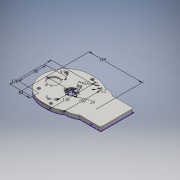
# Autodesk Inventor part: AZ-FLDIC-FWup bottom adapter
Saved by Autodesk Inventor 2016 (Build 200138000, 138)
## iProperties
Created: 2015-08-14
Part Number: AZ-FLDIC-FWup bottom adapter
Material: Generic
Document SubType Name: Modeling
Designer: kthorn
Density: 1 g/cm^3
Appearance: Default
Author: kthorn
Autodesk Inventor part; units mm, degrees
note: some values were not read from the file. Chosen so that the rebuilt part matches the saved one: sketch regions of "Extrusion4".
ref_plane "YZ Plane" through (0, 0, 0) normal (1, 0, 0) x (0, 1, 0)
ref_plane "XZ Plane" through (0, 0, 0) normal (0, 1, 0) x (-1, 0, 0)
ref_plane "XY Plane" through (0, 0, 0) normal (0, 0, 1) x (1, 0, 0)
sketch "Sketch1" plane through (0, 0, 0) normal (0, 0, 1) x (1, 0, 0)
  line L0 (-19.2849, 35) -> (-19.2849, -35) construction
  line L1 (19.7114, 54.5) -> (19.7114, -54.5) construction
  line L2 (-19.2849, 35) -> (19.7114, 54.5) construction
  line L3 (-19.2849, -35) -> (19.7114, -54.5) construction
  circle A0 centre (0.08, 0) radius 14.5
  line L4 (-19.2849, 35) -> (0.08, 0) construction
  line L5 (0.08, 0) -> (-19.2849, -35) construction
  circle A1 centre (19.7114, 54.5) radius 1.6 construction
  circle A2 centre (-19.2849, 35) radius 1.6 construction
  circle A3 centre (-19.2849, -35) radius 1.6 construction
  circle A4 centre (19.7114, -54.5) radius 1.6 construction
  line L6 (-16, -69) -> (0, -69)
  line L7 (0, 69) -> (-16, 69)
  arc A5 (-16, 69) -> (-16, -69) centre (-16, 0) ccw
  arc A6 (0, -69) -> (0, 69) centre (0, 0) ccw
  line L8 (-85, 0) -> (69, 0) construction
  circle A7 centre (-19.2849, 35) radius 3 construction
  circle A8 centre (-19.2849, -35) radius 3 construction
  circle A9 centre (19.7114, 54.5) radius 3 construction
  circle A10 centre (19.7114, -54.5) radius 3 construction
  line L9 (0.08, 60) -> (0.08, -60) construction
  line L10 (-55, -40) -> (-55, 40) construction
  circle A11 centre (-55, 40) radius 2.25
  circle A12 centre (-55, -40) radius 2.25
  circle A13 centre (0.08, -60) radius 2.25
  circle A14 centre (0.08, 60) radius 2.25
  point P0 (-19.2849, 0)
  point P1 (19.7114, 0)
  point P2 (-55, 0)
  dimension "d0" = 70
  dimension "d1" = 109
  dimension "d2" = 43.6
  dimension "d3" = 29
  dimension "d4" = 40
  dimension "d5" = 3.2
  dimension "d7" = 138
  dimension "d8" = 154
  dimension "d33" = 6
  dimension "d55" = 85.08
  dimension "d74" = 80
  dimension "d76" = 30
  dimension "d77" = 4.5
  dimension "d78" = 120
  constraints: 22 end point, 15 centre point, 13 coincident, 8 equal radius, 6 point on circle, 4 midpoint, 4 point on line, 3 equal length, 2 parallel, 2 tangent, 2 vertical, 1 horizontal
  measures "d0" distance of L0.start L0.end
  measures "d1" distance of L1.start L1.end
  measures "d2" distance of L0.start L1.start
  measures "d3" diameter of A0
  measures "d4" distance of L0.start L4.end
  measures "d5" diameter of A1
  measures "d7" distance of L7.end L6.start
  measures "d8" distance of L8.start L8.end
  measures "d33" diameter of A8
  measures "d55" distance of L4.end L8.start
  measures "d74" distance of L10.start L10.end
  measures "d76" distance from line of L10 L8.start
  measures "d77" diameter of A11
  measures "d78" distance of L9.start L9.end
extrude "Extrusion1" add sketch "Sketch1" along normal blind 11 contours A5 L7 A6 L6 | A11 | A12 | A13 | A14
sketch "Sketch2" plane through (0, 0, 11) normal (0, 0, 1) x (1, 0, 0)
  circle A0 centre (-52.47, 0) radius 18.5329 construction
  circle A1 centre (-71.0029, 0) radius 1.25
  circle A2 centre (-43.2035, 16.05) radius 1.25
  circle A3 centre (-43.2035, -16.05) radius 1.25
  circle A4 centre (0.08, 0) radius 14.5 projected
  line L0 (-16, -69) -> (0, -69) projected
  arc A5 (0, -69) -> (0, 69) centre (0, 0) ccw projected
  line L1 (0, 69) -> (-16, 69) projected
  arc A6 (-16, 69) -> (-16, -69) centre (-16, 0) ccw projected
  arc A7 (-16, 69) -> (-16, -69) centre (-16, 0) ccw construction
  line L2 (-85, 0) -> (69, 0) construction
  circle A8 centre (-43.2035, -16.05) radius 5
  circle A9 centre (-43.2035, 16.05) radius 5
  circle A10 centre (-71.0029, 0) radius 5
  circle A11 centre (-52.47, 0) radius 16.25
  line L3 (-53.47, -16.2192) -> (-53.47, -23.7192)
  line L4 (-53.47, -23.7192) -> (-51.47, -23.7192)
  line L5 (-51.47, -23.7192) -> (-51.47, -16.2192)
  line L6 (-52.47, -23.7192) -> (-52.47, 0) construction
  arc A12 (-53.47, -16.2192) -> (-51.47, -16.2192) centre (-52.47, 0) ccw
  dimension "d67" = 32.5
  dimension "d11" = 120
  dimension "d12" = 120
  dimension "d13" = 32.1
  dimension "d14" = 52.55
  dimension "d40" = 2.5
  dimension "d49" = 10
  dimension "d97" = 7.5
  dimension "d98" = 2
  constraints: 10 end point, 8 centre point, 8 point on circle, 5 coincident, 4 equal radius, 2 perpendicular, 2 point on line, 2 vertical, 1 midpoint, 1 parallel, 3 other
  measures "d13" distance of A2.centre A1.centre
  measures "d14" distance of A0.centre A4.centre
  measures "d40" diameter of A2
  measures "d49" diameter of A9
  measures "d97" distance of L3.start L3.end
  measures "d98" distance of L3.end L4.end
sketch "Sketch3" plane through (0, 0, 0) normal (0, 0, -1) x (-1, 0, 0)
  circle A0 centre (30.8533, 41.3) radius 6
  circle A1 centre (-0.08, 0) radius 14.5 projected
  circle A2 centre (30.8533, -41.3) radius 6
  line L0 (30.8533, 41.3) -> (-0.08, 0) construction
  line L1 (-0.08, 0) -> (30.8533, -41.3) construction
  circle A3 centre (-38.88, 0) radius 55.5
  circle A4 centre (-0.08, 0) radius 14.5 construction
  line L2 (16, -69) -> (0, -69) construction
  arc A5 (16, -69) -> (16, 69) centre (16, 0) ccw construction
  line L3 (0, 69) -> (16, 69) construction
  arc A6 (0, 69) -> (0, -69) centre (0, 0) ccw construction
  arc A7 (16, -69) -> (16, 69) centre (16, 0) ccw construction
  line L4 (85, 0) -> (-129.38, 0) construction
  arc A8 (0, 69) -> (0, -69) centre (0, 0) ccw construction
  line L5 (30.8533, 41.3) -> (30.8533, -41.3)
  line L6 (37.1783, 47.625) -> (-131.38, 47.625)
  line L7 (-131.38, 47.625) -> (-131.38, -47.625)
  line L8 (-131.38, -47.625) -> (37.1783, -47.625)
  line L9 (37.1783, -47.625) -> (37.1783, 47.625)
  line L10 (30.8533, 41.3) -> (37.1783, 41.3) construction
  line L11 (30.8533, 41.3) -> (30.8533, 47.625) construction
  line L12 (30.8533, -41.3) -> (37.1783, -41.3) construction
  line L13 (30.8533, -41.3) -> (30.8533, -47.625) construction
  circle A9 centre (-107.4467, 41.3) radius 6
  circle A10 centre (-107.4467, -41.3) radius 6
  line L14 (30.8533, 41.3) -> (-107.4467, 41.3) construction
  line L15 (30.8533, -41.3) -> (-107.4467, -41.3) construction
  circle A11 centre (-111.88, 0) radius 17.5
  line L16 (-111.88, 17.5) -> (-91.5488, 17.5)
  line L17 (-111.88, -17.5) -> (-91.5488, -17.5)
  circle A12 centre (-38.88, 0) radius 57.5
  line L18 (-131.38, 0) -> (-129.38, 0)
  line L19 (-111.88, 17.5) -> (-111.88, -17.5) construction
  line L20 (-113.4467, 41.3) -> (-113.4467, 47.625)
  line L21 (-101.4467, 41.3) -> (-101.4467, 47.625)
  line L22 (-113.4467, 41.3) -> (-101.4467, 41.3)
  line L23 (-113.4467, 47.625) -> (-101.4467, 47.625)
  line L24 (-113.4467, -41.3) -> (-113.4467, -47.625)
  line L25 (-113.4467, -47.625) -> (-101.4467, -47.625)
  line L26 (-101.4467, -47.625) -> (-101.4467, -41.3)
  line L27 (-101.4467, -41.3) -> (-113.4467, -41.3)
  dimension "d15" = 51.6
  dimension "d17" = 111
  dimension "d18" = 82.6
  dimension "d22" = 95.25
  dimension "d29" = 138.3
  dimension "d30" = 35
  dimension "d59" = 2
  dimension "d60" = 12
  dimension "d81" = 2
  dimension "d99" = 38.8
  constraints: 52 end point, 16 point on line, 11 point on circle, 7 centre point, 6 perpendicular, 5 horizontal, 4 equal length, 4 parallel, 3 collinear, 3 equal radius, 2 midpoint, 2 tangent, 2 vertical, 1 coincident
  measures "d15" distance of L0.end L0.start
  measures "d17" diameter of A3
  measures "d18" distance of L0.start L1.end
  measures "d22" distance of L6.end L7.end
  measures "d29" distance of L1.end L15.end
  measures "d30" diameter of A11
  measures "d59" radial gap between concentric circles of A12 A3
  measures "d60" diameter of A9
  measures "d81" distance of L18.start L4.end
  measures "d99" distance of L0.end A3.centre
extrude "Extrusion4" add sketch "Sketch3" against normal up to surface (11 mm away)
extrude "Extrusion14" cut sketch "Sketch3" against normal blind 6 contours A0 | A2 | L22 A9 | A9 L22 | L27 A10 | A10 L27
extrude "Extrusion15" cut sketch "Sketch3" against normal blind 10 contours A3 L6 L8 | A3 A11 A12 L16 | A11 A12 | A3 L17 A12 A11 | A3 L6 | A12 A11 L16 | A12 A11 | A12 L17 A11 | L8 A3
extrude "Extrusion16" cut sketch "Sketch2" against normal through all contours A1 | A2 | A3
extrude "Extrusion17" cut sketch "Sketch2" against normal blind 3 contours A11 A8 | A8 A11 A10 A9 | L5 L4 L3 A11 | A9 A11 | A11 A10 picked at (-44.8177, -13.2541) picked at (-44.8177, 13.2541) picked at (-67.7746, 0)
fillet "Fillet1" radius 5 1 edges at (131.38, -47.625, 5.5)
fillet "Fillet2" radius 5 1 edges at (131.38, 47.625, 5.5)
extrude "Extrusion20" cut sketch "Sketch1" along normal through all contours A11 | A12 | A13 | A14
sketch "Sketch10" plane through (0, 0, 11) normal (0, 0, 1) x (1, 0, 0)
  circle A0 centre (0.08, -60) radius 2.25 projected
  circle A1 centre (0.08, 60) radius 2.25 projected
  circle A2 centre (-55, 40) radius 2.25 projected
  circle A3 centre (-55, -40) radius 4
  circle A4 centre (0.08, -60) radius 4
  circle A5 centre (0.08, 60) radius 2.25 projected
  circle A6 centre (0.08, 60) radius 4
  circle A7 centre (-55, 40) radius 4
  point P0 (0, 0)
  dimension "d88" = 8
  constraints: 4 centre point, 4 coincident, 3 equal radius
  measures "d88" diameter of A3
extrude "Extrusion21" cut sketch "Sketch10" against normal blind 5
thread "Thread1" size "M3x0.5" class "6H" standard "ANSI Metric M Profile" full length
thread "Thread2" size "M3x0.5" class "6H" standard "ANSI Metric M Profile" full length
thread "Thread3" size "M3x0.5" class "6H" standard "ANSI Metric M Profile" full length
extrude "Extrusion22" cut sketch "Sketch3" against normal up to surface (6 mm away) contours L21 A9 L20 L6 | L8 L24 A10 L26
body "Solid1"
